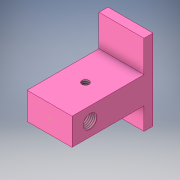
# Autodesk Inventor part: Support For Arms
Saved by Autodesk Inventor 2016 (Build 200138000, 138)
## iProperties
Created: 2015-07-13
Part Number: Support For Arms
Material: Aluminum 6061
Document SubType Name: Modeling
Designer: steele
Density: 2.7 g/cm^3
Appearance: Pink
Mass: 94.7579 g
Surface Area: 105.47 cm^2
Volume: 35.0955 cm^3
Author: steele
Autodesk Inventor part; units mm, degrees
ref_plane "YZ Plane" through (0, 0, 0) normal (1, 0, 0) x (0, 1, 0)
ref_plane "XZ Plane" through (0, 0, 0) normal (0, 1, 0) x (-1, 0, 0)
ref_plane "XY Plane" through (0, 0, 0) normal (0, 0, 1) x (1, 0, 0)
sketch "Sketch1" plane through (0, 0, 0) normal (0, 0, 1) x (1, 0, 0)
  line L0 (-15.875, -31.75) -> (15.875, -31.75)
  line L1 (15.875, -31.75) -> (15.875, 31.75)
  line L2 (15.875, 31.75) -> (-15.875, 31.75)
  line L3 (-15.875, 31.75) -> (-15.875, -31.75)
  line L4 (-15.875, -31.75) -> (15.875, 31.75) construction
  line L5 (15.875, -31.75) -> (-15.875, 31.75) construction
  point P0 (0, 0)
  dimension "height" = 63.5
  dimension "width" = 31.75
  constraints: 12 end point, 2 midpoint, 2 parallel, 1 horizontal, 1 perpendicular
  measures "height" distance of L0.end L1.end
  measures "width" distance of L1.end L2.end
extrude "Extrusion1" add sketch "Sketch1" against normal blind 12.7
sketch "Sketch3" plane through (0, 0, 0) normal (0, 0, 1) x (1, 0, 0)
  line L0 (-15.875, -9.525) -> (15.875, -9.525)
  line L1 (15.875, -9.525) -> (15.875, 9.525)
  line L2 (15.875, 9.525) -> (-15.875, 9.525)
  line L3 (-15.875, 9.525) -> (-15.875, -9.525)
  line L4 (-15.875, -9.525) -> (15.875, 9.525) construction
  line L5 (15.875, -9.525) -> (-15.875, 9.525) construction
  line L6 (15.875, 31.75) -> (-15.875, 31.75) projected
  point P0 (0, 0)
  dimension "Channel_Width" = 19.05
  dimension "d52" = 31.75
  constraints: 12 end point, 3 parallel, 2 midpoint, 1 perpendicular
  measures "Channel_Width" distance of L1.end L0.end
  measures "d52" distance of L1.end L2.end
extrude "Extrusion3" add sketch "Sketch3" along normal blind 50.8
sketch "Sketch6" plane through (15.875, -31.75, -12.7) normal (1, 0, 0) x (0, 0, -1)
  line L0 (-12.7, 31.75) -> (-63.5, 31.75) construction
  line L1 (-63.5, 22.225) -> (-63.5, 41.275) construction
  line L2 (-12.7, 41.275) -> (-12.7, 63.5) construction
  point P0 (-50.8, 31.75)
  dimension "d53" = 38.1
  constraints: 2 end point, 1 midpoint, 1 point on line
  measures "d53" distance from line of point (-50.8, 31.75) L2
hole "Hole5" at (15.875, 0, 38.1) direction (-1, 0, 0) diameter 9.7282 end through all thread size "7/16-20 UNF" class "2B" standard "ANSI Unified Screw Threads"
sketch "Sketch13" plane through (15.875, -31.75, -12.7) normal (1, 0, 0) x (0, 0, -1)
  line L0 (-12.7, 63.5) -> (0, 63.5) projected
  line L1 (0, 0) -> (-6.35, 0)
  line L2 (-6.35, 0) -> (-6.35, 63.5)
  line L3 (-6.35, 63.5) -> (0, 63.5)
  line L4 (0, 63.5) -> (0, 0)
  point P0 (-12.7, 31.75)
  dimension "d98" = 6.35
  constraints: 8 end point, 2 parallel, 1 horizontal, 1 midpoint, 1 perpendicular
  measures "d98" distance between parallel lines of L2 L4
extrude "Extrusion5" cut sketch "Sketch13" against normal through all
sketch "Sketch14" plane through (-15.875, -31.75, 0) normal (-1, 0, 0) x (0, 0, 1)
  line L0 (0, 0) -> (-6.35, 0) projected
  line L1 (0, 0) -> (0, 22.225) projected
  line L2 (-6.35, 0) -> (0, 0)
  line L3 (0, 0) -> (0, 6.604)
  line L4 (0, 6.604) -> (-6.35, 6.604)
  line L5 (-6.35, 6.604) -> (-6.35, 0)
  point P0 (0, 31.75)
  dimension "d101" = 6.604
  constraints: 8 end point, 2 parallel, 1 horizontal, 1 perpendicular, 1 point on line
  measures "d101" distance of L3.end L2.end
extrude "Extrusion6" cut sketch "Sketch14" against normal through all
sketch "Sketch15" plane through (-15.875, 9.525, 0) normal (0, 1, 0) x (1, 0, 0)
  line L0 (31.75, -50.8) -> (0, -50.8) projected
  point P0 (15.875, 0)
  point P1 (15.875, -25.4)
  dimension "d104" = 25.4
  measures "d104" distance from line of L0 point (15.875, -25.4)
hole "Hole11" at (0, 9.525, 25.4) direction (0, -1, 0) diameter 4.9784 end through all thread size "1/4-20 UNC" class "2B" standard "ANSI Unified Screw Threads"
sketch "Sketch10" plane through (0, 0, 50.8) normal (0, 0, 1) x (1, 0, 0)
  point P0 (0, 0)
sketch "Sketch11" plane through (0, 0, 50.8) normal (0, 0, 1) x (1, 0, 0)
  point P0 (0, 0)
sketch "Sketch12" plane through (-15.875, -9.525, 0) normal (0, -1, 0) x (1, 0, 0)
  point P0 (15.875, 15.875)
equation "\"d52\" = width"
body "Solid1"
